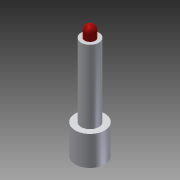
# Autodesk Inventor part: Lilin
Saved by Autodesk Inventor 2015 (Build 190159000, 159)
## iProperties
Created: 2012-11-29
Part Number: Lilin
Material: Generic
Document SubType Name: Modeling
Designer: irwan
Density: 1 g/cm^3
Appearance: Cool White
Author: irwan
Autodesk Inventor part; units mm, degrees
ref_plane "YZ Plane" through (0, 0, 0) normal (1, 0, 0) x (0, 1, 0)
ref_plane "Work Plane1" through (0, 0, 4) normal (0, 0, 1) x (1, 0, 0)
sketch "Sketch2" plane through (0, 0, 4) normal (0, 0, 1) x (1, 0, 0)
  circle A0 centre (0, 0) radius 300 projected
  circle A1 centre (0, 0) radius 25
  circle A2 centre (0, 0) radius 15
  dimension "d3" = 50
  dimension "d4" = 30
  constraints: 2 centre point, 2 coincident
  measures "d3" diameter of A1
  measures "d4" diameter of A2
extrude "Extrusion2" add sketch "Sketch2" along normal blind 50 contours A1 | A2
extrude "Extrusion3" add sketch "Sketch2" along normal blind 174 contours A2
ref_plane "Work Plane3" through (0, 0, 178) normal (0, 0, 1) x (1, 0, 0)
sketch "Sketch3" plane through (0, 0, 178) normal (0, 0, 1) x (1, 0, 0)
  circle A0 centre (0, 0) radius 15 projected
  circle A1 centre (0, 0) radius 9
  dimension "d9" = 18
  constraints: 1 centre point, 1 coincident
  measures "d9" diameter of A1
extrude "Extrusion4" add sketch "Sketch3" along normal blind 20 contours A1
ref_plane "Work Plane2" through (0, 0, 4) normal (0, 0, 1) x (1, 0, 0)
sketch "Sketch4" plane through (0, 0, 4) normal (0, 0, 1) x (1, 0, 0)
  circle A0 centre (0, 0) radius 25 projected
  circle A1 centre (0, 0) radius 300 projected
  line L0 (0, 0) -> (0, 300)
  line L1 (0, 0) -> (0, -300)
  line L2 (0, 0) -> (300, 0)
  constraints: 6 end point, 3 point on circle, 1 collinear, 1 perpendicular, 1 vertical
fillet "Fillet2" radius 9 1 edges at (-9, 0, 198)
body "Solid1"
